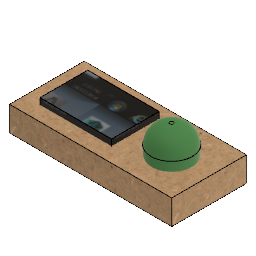
button and screen (Autodesk Fusion 360 design; units mm, degrees)
Autodesk Fusion 360 part; units mm, degrees
sketch "Esquisse1" plane through (0, 0, 0) normal (0, 0, 1) x (1, 0, 0)
  line L0 (-20, 60) -> (-77.288, 60)
  line L1 (-77.288, 60) -> (-77.288, 21.808)
  line L2 (-77.288, 21.808) -> (-20, 21.808)
  line L3 (-20, 21.808) -> (-20, 60)
  dimension "d1" = 57.288
  dimension "d2" = 38.192
  constraint horizontal L0
  constraint vertical L1
  constraint horizontal L2
  constraint vertical L3
  measures "d1" distance of L0.start L0.end
  measures "d2" distance of L0.start L2.end
sketch "Esquisse2" plane through (0, 0, 0) normal (0, 0, 1) x (1, 0, 0)
  circle A0 centre (10, 40) radius 16.5
  dimension "d3" = 33
  measures "d3" diameter of A0
sketch "Esquisse3" plane through (0, 0, 0) normal (0, 0, 1) x (1, 0, 0)
  line L0 (-90, 70) -> (40, 70)
  line L1 (40, 70) -> (40, 10)
  line L2 (40, 10) -> (-90, 10)
  line L3 (-90, 10) -> (-90, 70)
  constraint horizontal L0
  constraint vertical L1
  constraint horizontal L2
  constraint vertical L3
extrude "Extrusion1" add sketch "Esquisse2" along normal blind 42 makes body 1
extrude "Extrusion2" add sketch "Esquisse1" along normal blind 25 separate body makes body 2
extrude "Extrusion3" add sketch "Esquisse3" along normal blind 20 separate body makes body 3
fillet "Congé1" radius 15 1 edges at (-5.3834, 34.0333, 42) on bodies 1
